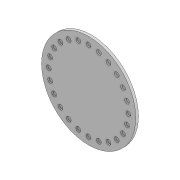
# Autodesk Inventor part: pindisk
Saved by Autodesk Inventor 2022 (Build 260153000, 153)
## iProperties
Created: 2023-11-18
Part Number: pindisk
Material: 一般
Document SubType Name: Modeling
Designer: JOU
Density: 1 g/cm^3
Appearance: 預設
Author: JOU
Autodesk Inventor part; units mm, degrees
ref_plane "YZ Plane" through (0, 0, 0) normal (1, 0, 0) x (0, 1, 0)
ref_plane "XZ Plane" through (0, 0, 0) normal (0, 1, 0) x (-1, 0, 0)
ref_plane "XY Plane" through (0, 0, 0) normal (0, 0, 1) x (1, 0, 0)
sketch "草圖2" plane through (0, 0, 0) normal (0, 0, 1) x (1, 0, 0)
  circle A0 centre (0, 0) radius 177.5
  dimension "d8" = 355
  constraints: 1 centre point, 1 coincident
  measures "d8" diameter of A0
extrude "擠出2" add sketch "草圖2" against normal blind 10
sketch "草圖1" plane through (0, 0, 0) normal (0, 0, 1) x (1, 0, 0)
  circle A0 centre (150, 0) radius 9
  circle A1 centre (144.8889, 38.8229) radius 9
  circle A2 centre (129.9038, 75) radius 9
  circle A3 centre (106.066, 106.066) radius 9
  circle A4 centre (75, 129.9038) radius 9
  circle A5 centre (38.8229, 144.8889) radius 9
  circle A6 centre (0, 150) radius 9
  circle A7 centre (-38.8229, 144.8889) radius 9
  circle A8 centre (-75, 129.9038) radius 9
  circle A9 centre (-106.066, 106.066) radius 9
  circle A10 centre (-129.9038, 75) radius 9
  circle A11 centre (-144.8889, 38.8229) radius 9
  circle A12 centre (-150, 0) radius 9
  circle A13 centre (-144.8889, -38.8229) radius 9
  circle A14 centre (-129.9038, -75) radius 9
  circle A15 centre (-106.066, -106.066) radius 9
  circle A16 centre (-75, -129.9038) radius 9
  circle A17 centre (-38.8229, -144.8889) radius 9
  circle A18 centre (0, -150) radius 9
  circle A19 centre (38.8229, -144.8889) radius 9
  circle A20 centre (75, -129.9038) radius 9
  circle A21 centre (106.066, -106.066) radius 9
  circle A22 centre (129.9038, -75) radius 9
  circle A23 centre (144.8889, -38.8229) radius 9
  point P0 (0, 0)
  dimension "d0" = 150
  dimension "d1" = 18
  dimension "d4" = 360
  constraints: 24 centre point, 1 horizontal alignment, 49 other
  measures "d0" distance of point (0, 0) A0.centre
  measures "d1" diameter of A0
extrude "擠出3" cut sketch "草圖1" against normal blind 5
